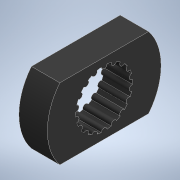
# Autodesk Inventor part: Rubber
Saved by Autodesk Inventor 2021 (Build 250183000, 183)
## iProperties
Created: 2021-03-23
Part Number: Rubber
Material: Generic
Document SubType Name: Modeling
Designer: calst
Density: 1 g/cm^3
Appearance: Rubber - Black
Author: calst
Autodesk Inventor part; units mm, degrees
ref_plane "YZ Plane" through (0, 0, 0) normal (1, 0, 0) x (0, 1, 0)
ref_plane "XZ Plane" through (0, 0, 0) normal (0, 1, 0) x (-1, 0, 0)
ref_plane "XY Plane" through (0, 0, 0) normal (0, 0, 1) x (1, 0, 0)
sketch "Sketch1" plane through (0, 0, 0) normal (1, 0, 0) x (0, 1, 0)
  circle A0 centre (0, 0) radius 10
  line L0 (12.5, 0) -> (12.5, -15.6125)
  line L1 (12.5, 0) -> (12.5, 15.6125)
  line L2 (-12.5, 0) -> (-12.5, -15.6125)
  line L3 (-12.5, 0) -> (-12.5, 15.6125)
  arc A1 (12.5, 15.6125) -> (-12.5, 15.6125) centre (0, 0) ccw
  arc A2 (-12.5, -15.6125) -> (12.5, -15.6125) centre (0, 0) ccw
  dimension "d0" = 20
  constraints: 8 end point, 4 point on circle, 3 centre point, 2 coincident, 2 point on line
  measures "d0" diameter of A0
extrude "Extrusion1" add sketch "Sketch1" along normal blind 10
sketch "Sketch2" plane through (10, 0, 0) normal (1, 0, 0) x (0, 0, -1)
  circle A0 centre (0, 0) radius 10 projected
  circle A1 centre (0, 10) radius 1
  circle A2 centre (-3.4202, 9.3969) radius 1
  circle A3 centre (-6.4279, 7.6604) radius 1
  circle A4 centre (-8.6603, 5) radius 1
  circle A5 centre (-9.8481, 1.7365) radius 1
  circle A6 centre (-9.8481, -1.7365) radius 1
  circle A7 centre (-8.6603, -5) radius 1
  circle A8 centre (-6.4279, -7.6604) radius 1
  circle A9 centre (-3.4202, -9.3969) radius 1
  circle A10 centre (0, -10) radius 1
  circle A11 centre (3.4202, -9.3969) radius 1
  circle A12 centre (6.4279, -7.6604) radius 1
  circle A13 centre (8.6603, -5) radius 1
  circle A14 centre (9.8481, -1.7365) radius 1
  circle A15 centre (9.8481, 1.7365) radius 1
  circle A16 centre (8.6603, 5) radius 1
  circle A17 centre (6.4279, 7.6604) radius 1
  circle A18 centre (3.4202, 9.3969) radius 1
  dimension "d6" = 2
  dimension "d9" = 360
  constraints: 18 centre point, 1 vertical alignment, 38 other
  measures "d6" diameter of A1
extrude "Extrusion2" add sketch "Sketch2" against normal blind 10 contours A15 A0 | A0 A15 | A14 A0 | A0 A14 | A16 A0 | A0 A16 | A13 A0 | A0 A13 | A17 A0 | A0 A17 | A12 A0 | A0 A12 | A18 A0 | A0 A18 | A11 A0 | A0 A11 | A1 A0 | A0 A1 | A10 A0 | A0 A10 | A2 A0 | A0 A2 | A9 A0 | A0 A9 | A3 A0 | A0 A3 | A8 A0 | A0 A8 | A4 A0 | A0 A4 | A7 A0 | A0 A7 | A5 A0 | A0 A5 | A6 A0 | A0 A6
body "Solid1"
